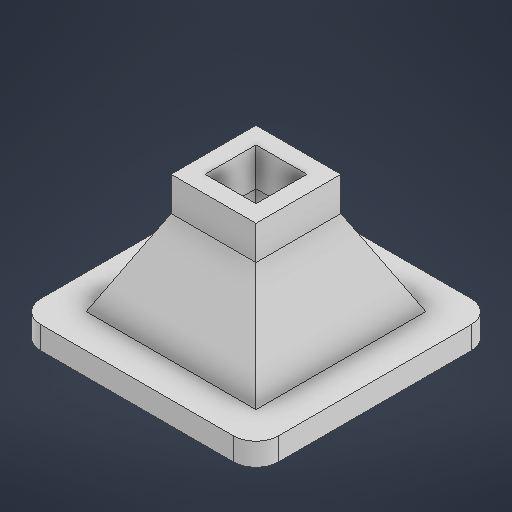
# Autodesk Inventor part: ejercicio_clase_5
Saved by Autodesk Inventor 2026.1 (Build 301233020, 233B)
## iProperties
Created: 2026-02-07
Part Number: ejercicio_clase_5
Material: Genérico
Document SubType Name: Modeling
Designer: UPN
Density: 1 g/cm^3
Appearance: Valor por defecto
Author: UPN
Autodesk Inventor part; units mm, degrees
ref_plane "YZ Plane" through (0, 0, 0) normal (1, 0, 0) x (0, 1, 0)
ref_plane "XZ Plane" through (0, 0, 0) normal (0, 1, 0) x (-1, 0, 0)
sketch "Boceto1" plane through (0, 0, 0) normal (0, 1, 0) x (-1, 0, 0)
  line L0 (-2.125, 2.625) -> (2.125, 2.625)
  line L1 (2.625, 2.125) -> (2.625, -2.125)
  line L2 (2.125, -2.625) -> (-2.125, -2.625)
  line L3 (-2.625, -2.125) -> (-2.625, 2.125)
  line L4 (-2.625, 2.625) -> (2.625, -2.625) construction
  line L5 (2.625, 2.625) -> (-2.625, -2.625) construction
  arc A0 (2.625, 2.125) -> (2.125, 2.625) centre (2.125, 2.125) ccw
  arc A1 (2.125, -2.625) -> (2.625, -2.125) centre (2.125, -2.125) ccw
  arc A2 (-2.625, -2.125) -> (-2.125, -2.625) centre (-2.125, -2.125) ccw
  arc A3 (-2.125, 2.625) -> (-2.625, 2.125) centre (-2.125, 2.125) ccw
  point P0 (0, 0)
  point P1 (0, -2.625)
  dimension "d0" = 0.5
  dimension "d1" = 5.25
  dimension "d2" = 5.25
  constraints: 12 end point, 8 point on circle, 8 point on line, 8 tangent, 4 centre point, 3 equal radius, 3 midpoint, 2 parallel, 1 horizontal, 1 perpendicular
  measures "d0" radius of A0
  measures "d1" distance between parallel lines of L3 L1
  measures "d2" distance from line of point (0, -2.625) L0
extrude "Extrusión1" add sketch "Boceto1" along normal blind 0.5
sketch "Boceto2" plane through (0, 0.5, 0) normal (0, 1, 0) x (1, 0, 0)
  line L0 (1.875, -1.875) -> (-1.875, -1.875)
  line L1 (-1.875, -1.875) -> (-1.875, 1.875)
  line L2 (-1.875, 1.875) -> (1.875, 1.875)
  line L3 (1.875, 1.875) -> (1.875, -1.875)
  line L4 (1.875, -1.875) -> (-1.875, 1.875) construction
  line L5 (-1.875, -1.875) -> (1.875, 1.875) construction
  point P0 (0, 0)
  dimension "d5" = 3.75
  dimension "d6" = 3.75
  constraints: 12 end point, 2 midpoint, 2 parallel, 1 horizontal, 1 perpendicular
  measures "d5" distance of L0.end L1.end
  measures "d6" distance of L0.start L0.end
ref_plane "Plano de trabajo1" through (0, 2.375, 0) normal (0, 1, 0) x (1, 0, 0)
sketch "Boceto3" plane through (0, 2.375, 0) normal (0, 1, 0) x (1, 0, 0)
  line L0 (0.9375, -0.9375) -> (-0.9375, -0.9375)
  line L1 (-0.9375, -0.9375) -> (-0.9375, 0.9375)
  line L2 (-0.9375, 0.9375) -> (0.9375, 0.9375)
  line L3 (0.9375, 0.9375) -> (0.9375, -0.9375)
  line L4 (0.9375, -0.9375) -> (-0.9375, 0.9375) construction
  line L5 (-0.9375, -0.9375) -> (0.9375, 0.9375) construction
  point P0 (0, 0)
  dimension "d8" = 1.875
  dimension "d9" = 1.875
  constraints: 12 end point, 2 midpoint, 2 parallel, 1 horizontal, 1 perpendicular
  measures "d8" distance of L0.end L1.end
  measures "d9" distance of L1.end L2.end
loft "Solevación1" add profiles "Boceto2", "Boceto3"
sketch "Boceto4" plane through (-0.9375, 2.375, 0.9375) normal (0, 1, 0) x (1, 0, 0)
  line L0 (1.875, 0) -> (0, 0) projected
  line L1 (1.875, 1.875) -> (1.875, 0) projected
  line L2 (0, 1.875) -> (1.875, 1.875) projected
  line L3 (0, 0) -> (0, 1.875) projected
  point P0 (0.9375, 0.9375)
extrude "Extrusión2" add sketch "Boceto4" along normal blind 0.75
shell "Vaciado5" thickness 0.375 removed faces 1 at (0.3125, 3.125, 0.3125)
sketch "Boceto11" plane through (0, 0, 0) normal (0, 0, 1) x (1, 0, 0)
  line L0 (1.5182, 0.375) -> (0.5625, 2.2865) projected
  line L1 (-1.5182, 0.375) -> (-0.5625, 2.2865) projected
  line L2 (1.5182, 0.375) -> (1.7057, 0)
  line L3 (-1.5182, 0.375) -> (-1.7057, 0)
  line L4 (1.7057, 0) -> (-1.7057, 0)
  point P0 (0, 0)
  point P1 (-2.625, 0)
  constraints: 6 end point, 2 collinear, 1 horizontal, 1 horizontal alignment
sketch "Boceto10" plane through (0, 0, 0) normal (0, -1, 0) x (1, 0, 0)
  line L0 (1.7057, 1.7057) -> (-1.7057, 1.7057)
  line L1 (-1.7057, 1.7057) -> (-1.7057, -1.7057)
  line L2 (-1.7057, -1.7057) -> (1.7057, -1.7057)
  line L3 (1.7057, -1.7057) -> (1.7057, 1.7057)
  line L4 (1.7057, 1.7057) -> (-1.7057, -1.7057) construction
  line L5 (-1.7057, 1.7057) -> (1.7057, -1.7057) construction
  point P0 (0, 0)
  point P1 (-1.7057, 0)
  point P2 (-1.7057, 0)
  constraints: 12 end point, 3 midpoint, 2 parallel, 2 perpendicular, 1 coincident, 1 horizontal
sketch "Boceto12" plane through (-1.5182, 0.375, -1.5182) normal (0, 1, 0) x (1, 0, 0)
  line L0 (3.0365, -3.0365) -> (3.0365, 0) projected
  line L1 (3.0365, 0) -> (0, 0) projected
  line L2 (0, 0) -> (0, -3.0365) projected
  line L3 (0, -3.0365) -> (3.0365, -3.0365) projected
  point P0 (1.5182, -1.5182)
loft "Solevación3" cut profiles "Boceto10" section 1 edges at (1.5182, 0.375, 0) (0, 0.375, -1.5182) (-1.5182, 0.375, 0) (0, 0.375, 1.5182)
equation "\"d2\" = d1"
equation "\"d6\" = d5"
equation "\"d9\" = d8"
